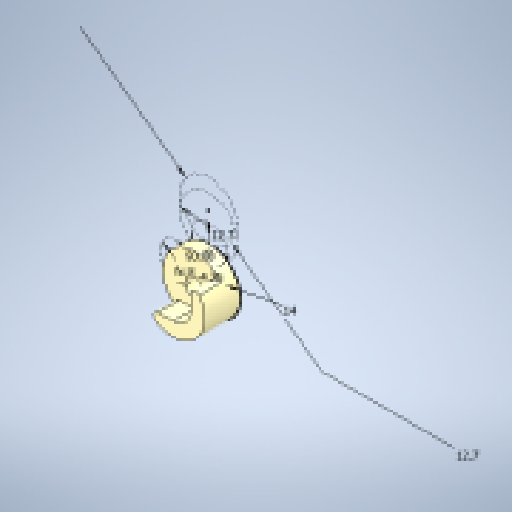
# Autodesk Inventor part: Cam - Shell
Saved by Autodesk Inventor 2023.2 (Build 272271000, 271)
## iProperties
Created: 2024-01-19
Part Number: Cam - Shell
Material: Nylon 6/6
Document SubType Name: Modeling
Designer: Nathan Cai
Density: 1.13 g/cm^3
Appearance: Nylon 6
Author: Nathan Cai
Autodesk Inventor part; units mm, degrees
ref_plane "YZ Plane" through (0, 0, 0) normal (1, 0, 0) x (0, 1, 0)
ref_plane "XZ Plane" through (0, 0, 0) normal (0, 1, 0) x (-1, 0, 0)
ref_plane "XY Plane" through (0, 0, 0) normal (0, 0, 1) x (1, 0, 0)
sketch "Sketch1" plane through (0, 0, 0) normal (0, 0, 1) x (1, 0, 0)
  circle A0 centre (0, 0) radius 2.125
  circle A1 centre (0, 0) radius 7
  line L0 (0, 0) -> (0, 7) construction
  line L1 (4, 0) -> (4, 7)
  line L2 (-4, 7) -> (-4, 0)
  arc A2 (-4, 0) -> (4, 0) centre (0, 0) ccw
  arc A3 (4, 7) -> (-4, 7) centre (0, 7) ccw construction
  line L3 (0, 0) -> (-7, 0) construction
  line L4 (0, 4) -> (-7, 4)
  line L5 (-7, -4) -> (0, -4)
  arc A4 (0, -4) -> (0, 4) centre (0, 0) ccw
  arc A5 (-7, 4) -> (-7, -4) centre (-7, 0) ccw construction
  circle A6 centre (0, 13.35) radius 6.35 construction
  circle A7 centre (0, 10.35) radius 6.35 construction
  point P0 (0, 3.5)
  point P1 (-3.5, 0)
  point P2 (0, -4)
  point P3 (-5.7446, -4)
  point P4 (4, 5.7446)
  dimension "d0" = 4.25
  dimension "d3" = 14
  dimension "d4" = 8
  dimension "d5" = 8
  dimension "d6" = 90
  dimension "d7" = 12.7
  dimension "d8" = 12.7
  constraints: 16 end point, 10 point on circle, 10 tangent, 8 centre point, 2 coincident, 2 midpoint, 2 parallel, 2 point on line, 1 vertical
  measures "d0" diameter of A0
  measures "d3" diameter of A1
  measures "d4" diameter of A3
  measures "d5" diameter of A5
  measures "d6" angle of L0 L3
  measures "d7" diameter of A6
  measures "d8" diameter of A7
extrude "Extrusion1" add sketch "Sketch1" along normal blind 3.175
extrude "Extrusion2" add sketch "Sketch1" along normal blind 7.9375 contours A1 L5 A2 L1
fillet "Fillet1" radius 1 2 edges at (4, 5.7446, 5.5563) (-5.7446, -4, 5.5563)
equation "\"d5\" = d4"
body "Solid1"
